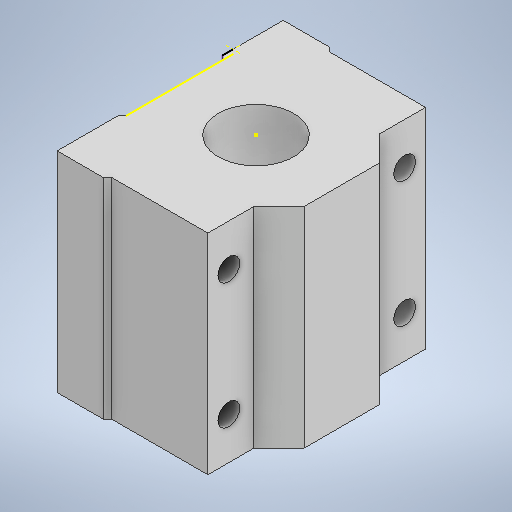
# Autodesk Inventor part: lozysko
Saved by Autodesk Inventor 2025 (Build 290162000, 162)
## iProperties
Created: 2024-04-05
Part Number: lozysko
Material: Generic
Document SubType Name: Modeling
Designer: Wojtek
Density: 1 g/cm^3
Appearance: Default
Author: Wojtek
Autodesk Inventor part; units mm, degrees
ref_plane "YZ Plane" through (0, 0, 0) normal (1, 0, 0) x (0, 1, 0)
ref_plane "XZ Plane" through (0, 0, 0) normal (0, 1, 0) x (-1, 0, 0)
ref_plane "XY Plane" through (0, 0, 0) normal (0, 0, 1) x (1, 0, 0)
sketch "Sketch1" plane through (0, 0, 0) normal (0, 1, 0) x (-1, 0, 0)
  circle A0 centre (0, 0) radius 9
  line L0 (-20.5, -27) -> (20.5, -27)
  line L1 (20.5, -27) -> (20.5, 27)
  line L2 (20.5, 27) -> (-20.5, 27)
  line L3 (-20.5, 27) -> (-20.5, -27)
  line L4 (-20.5, -27) -> (20.5, 27) construction
  line L5 (20.5, -27) -> (-20.5, 27) construction
  line L6 (-20.5, 9) -> (-15.1202, 14.3798)
  line L7 (-20.5, 9) -> (-12.8918, 9) construction
  line L8 (-15.1202, 14.3798) -> (-14.5001, 14.9999)
  line L9 (-14.5001, 14.9999) -> (-14.5001, 27)
  line L10 (20.5, 0) -> (-20.5, 0)
  line L11 (-20.5, -9) -> (-15.1202, -14.3798)
  line L12 (-15.1202, -14.3798) -> (-14.5001, -14.9999)
  line L13 (-14.5001, -14.9999) -> (-14.5001, -27)
  line L14 (9.5, 27) -> (12.281, 27) construction
  line L15 (9.5, 27) -> (8.5, 26)
  line L16 (9.5, 27) -> (10.9142, 27) construction
  line L17 (8.5, 26) -> (-14.5001, 26)
  line L18 (20.5, 15) -> (19.5, 14)
  line L19 (20.5, 15) -> (21.9142, 15) construction
  line L20 (19.5, 14) -> (19.5, 0)
  line L21 (9.5, -27) -> (8.5, -26)
  line L22 (8.5, -26) -> (-14.5001, -26)
  line L23 (20.5, -15) -> (19.5, -14)
  line L24 (19.5, -14) -> (19.5, 0)
  point P0 (0, 9)
  point P1 (0, 9)
  point P2 (19.5, 27)
  dimension "d0" = 18
  dimension "d1" = 41
  dimension "d2" = 54
  dimension "d4" = 45
  constraints: 50 end point, 9 point on line, 9 symmetric about line, 5 horizontal, 4 midpoint, 3 coincident, 3 equal length, 3 perpendicular, 2 parallel, 2 vertical alignment, 1 vertical, 2 other
  measures "d1" distance of L2.end L1.end
  measures "d2" distance of L1.end L0.end
  measures "d4" angle of L7 L6
extrude "Extrusion1" add sketch "Sketch1" along normal blind 50 contours L10 L24 L23 L1 L0 L21 L22 L13 L12 L11 L3 A0 | A0 L10 L3 L6 L8 L9 L17 L15 L2 L1 L18 L20
sketch "Sketch2" plane through (14.5001, 0, 26) normal (1, 0, 0) x (0, 0, -1)
  point P0 (26, 0)
sketch "Sketch3" plane through (-20.5, 0, 15) normal (-1, 0, 0) x (0, 0, 1)
  circle A0 centre (-36, 40) radius 3
  line L0 (-42, 0) -> (-42, 50) projected
  line L1 (-42, 25) -> (12, 25) construction
  circle A1 centre (-36, 10) radius 3
  line L2 (-24, 50) -> (-6, 50) projected
  circle A2 centre (6, 40) radius 3
  circle A3 centre (6, 10) radius 3
  point P0 (-15, 0)
  point P1 (-15, 25)
  dimension "d17" = 6
  constraints: 4 centre point, 2 end point, 1 horizontal, 1 midpoint
  measures "d17" diameter of A0
sketch "Sketch4" plane through (0, 0, 0) normal (0, -1, 0) x (1, 0, 0)
  line L0 (-19.5, -14) -> (-19.5, 14) projected
  line L1 (-19.5, 11.5) -> (-17.4106, 11.5) construction
  line L2 (-19.5, 14) -> (-20.5, 15) projected
  line L3 (-19.5, 11.5) -> (-20.3656, 12.3656)
  line L4 (-19.5, 11.5) -> (-18.2759, 11.5) construction
  line L5 (-20.3656, 12.3656) -> (-20.5, 12.5)
  line L6 (-20.5, 15) -> (-20.5, 12.5)
  line L7 (20.5, 9) -> (20.5, -9) projected
  line L8 (20.5, 0) -> (-19.5, 0)
  line L9 (-19.5, -11.5) -> (-20.3656, -12.3656)
  line L10 (-20.3656, -12.3656) -> (-20.5, -12.5)
  line L11 (-20.5, -15) -> (-20.5, -12.5)
  point P0 (0, 0)
  dimension "d12" = 135
  constraints: 18 end point, 4 symmetric about line, 3 point on line, 2 horizontal, 2 midpoint, 1 coincident, 1 equal length, 1 vertical
  measures "d12" angle of L4 L3
extrude "Extrusion2" add sketch "Sketch4" against normal blind 50
sketch "Sketch5" plane through (0, 50, 0) normal (0, 1, 0) x (1, 0, 0)
  point P0 (0, 0)
sketch "Sketch6" plane through (0, 50, 0) normal (0, 1, 0) x (1, 0, 0)
  line L0 (-20.5, 15) -> (-20.5, 12.5)
  line L1 (-20.5, 12.5) -> (-19.5, 11.5)
  line L2 (-19.5, 14) -> (-19.5, -11.5) projected
  point P0 (0, 0)
  constraints: 4 end point, 1 point on line, 1 vertical
mirror "Mirror1" about plane through (0, 0, 0) normal (0, 0, 1) of "Extrusion1"
mirror "Mirror2" about plane through (0, 0, 0) normal (0, 0, 1)
hole "Hole1" at (-20.5, 40, -21) at (-20.5, 10, -21) at (-20.5, 10, 21) at (-20.5, 40, 21) direction (1, 0, 0) diameter 5.2 end through all counterbore diameter 6 counterbore depth 12
body "Solid1"
